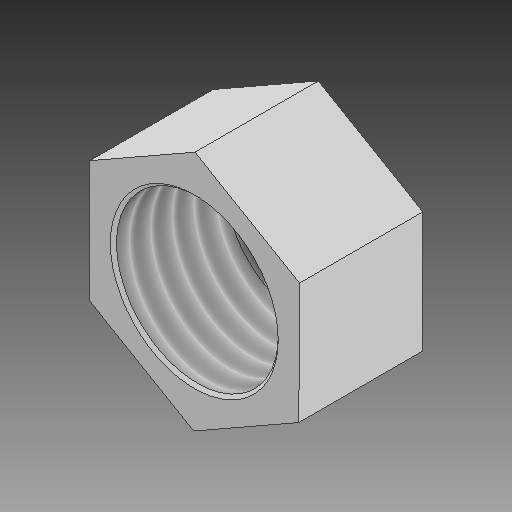
# Autodesk Inventor part: VerteilerLuft2
Saved by Autodesk Inventor 2021 (Build 250183000, 183)
## iProperties
Created: 2021-10-22
Part Number: VerteilerLuft2
Material: Generisch
Document SubType Name: Modeling
Designer: lukas
Density: 1 g/cm^3
Appearance: Vorgabe
Stock Number: Verteiler 2
Author: lukas
Autodesk Inventor part; units mm, degrees
ref_plane "YZ Plane" through (0, 0, 0) normal (1, 0, 0) x (0, 1, 0)
ref_plane "XZ Plane" through (0, 0, 0) normal (0, 1, 0) x (-1, 0, 0)
ref_plane "XY Plane" through (0, 0, 0) normal (0, 0, 1) x (1, 0, 0)
sketch "Skizze1" plane through (0, 0, 0) normal (0, 0, 1) x (1, 0, 0)
  line L0 (-23.874, 0) -> (23.874, 0) projected
  line L1 (0, -27.4815) -> (0, 27.4815) projected
  line L2 (-16.9467, 9.9068) -> (0.1062, 19.6296)
  line L3 (0.1062, 19.6296) -> (17.0529, 9.7228)
  line L4 (17.0529, 9.7228) -> (16.9467, -9.9068)
  line L5 (16.9467, -9.9068) -> (-0.1062, -19.6296)
  line L6 (-0.1062, -19.6296) -> (-17.0529, -9.7228)
  line L7 (-17.0529, -9.7228) -> (-16.9467, 9.9068)
  circle A0 centre (0, 0) radius 15
  dimension "d0" = 30
  dimension "d1" = 17
  constraints: 12 end point, 2 coincident, 1 centre point, 13 other
  measures "d0" diameter of A0
  measures "d1" distance from line of L4 A0.centre
extrude "Extrusion1" add sketch "Skizze1" along normal blind 20
sketch "Skizze3" plane through (0, 0, 20) normal (0, 0, 1) x (1, 0, 0)
  point P0 (0, 0)
hole "Bohrung1" at (0, 0, 20) direction (0, 0, -1) diameter 26.211 depth 18 thread size "M30x3.5" class "6H" standard "ISO Metric profile"
chamfer "Fase1" distance 0.5 angle 45 1 edges at (0, 13.1055, 20)
